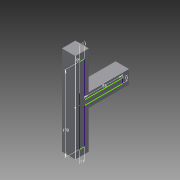
# Autodesk Inventor part: Main
Saved by Autodesk Inventor 2015 (Build 190159000, 159)
## iProperties
Created: 2015-06-22
Part Number: Main
Material: 一般
Document SubType Name: Modeling
Designer: hyt
Density: 1 g/cm^3
Appearance: 既定
Author: hyt
Autodesk Inventor part; units mm, degrees
ref_plane "YZ Plane" through (0, 0, 0) normal (1, 0, 0) x (0, 1, 0)
ref_plane "XZ Plane" through (0, 0, 0) normal (0, 1, 0) x (-1, 0, 0)
ref_plane "XY Plane" through (0, 0, 0) normal (0, 0, 1) x (1, 0, 0)
sketch "スケッチ1" plane through (0, 0, 0) normal (1, 0, 0) x (0, 1, 0)
  line L0 (30, 15) -> (120, 15)
  line L1 (120, 15) -> (120, -15)
  line L2 (120, -15) -> (30, -15)
  line L3 (0, -15) -> (0, 15)
  line L4 (30, 100) -> (0, 100)
  line L5 (0, 100) -> (0, -100)
  line L6 (0, -100) -> (30, -100)
  line L7 (30, -100) -> (30, -15)
  line L8 (30, 15) -> (30, 100)
  point P0 (0, 0)
  point P1 (0, 0)
  dimension "d0" = 30
  dimension "d1" = 120
  dimension "d2" = 30
  dimension "d3" = 200
  constraints: 18 end point, 4 parallel, 2 horizontal, 2 midpoint, 2 perpendicular, 1 coincident, 1 point on line
  measures "d0" distance of L0.end L1.end
  measures "d1" distance of L3.end L0.end
  measures "d2" distance of L5.end L6.end
  measures "d3" distance of L4.end L5.end
extrude "押し出し1" add sketch "スケッチ1" along normal blind 30
sketch "スケッチ2" plane through (30, 0, 0) normal (1, 0, 0) x (0, 0, -1)
  line L0 (-23.0571, 9) -> (23.0571, 9)
  line L1 (5.5, 20) -> (5.5, 105)
  line L2 (5.5, 105) -> (-5.5, 105)
  line L3 (-5.5, 105) -> (-5.5, 20)
  line L4 (-100, 0) -> (100, 0) projected
  line L5 (-85, 9) -> (85, 9)
  line L6 (85, 9) -> (85, 20)
  line L7 (-85, 20) -> (-85, 9)
  line L8 (85, 20) -> (5.5, 20)
  line L9 (-5.5, 20) -> (-85, 20)
  point P0 (0, 0)
  point P1 (0, 9)
  dimension "d6" = 11
  dimension "d8" = 11
  dimension "d9" = 170
  dimension "d10" = 9
  dimension "d11" = 11
  dimension "d12" = 85
  constraints: 18 end point, 5 parallel, 2 horizontal, 2 midpoint, 2 perpendicular
  measures "d6" distance of L1.end L2.end
  measures "d8" distance of L5.end L6.end
  measures "d9" distance of L5.start L5.end
  measures "d10" distance from line of L0.start L4
  measures "d11" distance of L7.start L5.start
  measures "d12" distance of L2.end L3.end
sketch "スケッチ3" plane through (30, 0, 0) normal (1, 0, 0) x (0, 0, -1)
  point P0 (0, 0)
equation "\"d11\" = d8"
